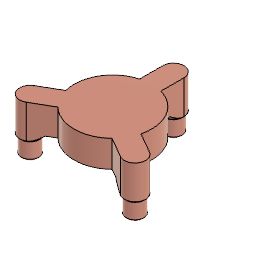
CarrierGenerator (Autodesk Fusion 360 design; units mm, degrees)
Autodesk Fusion 360 part; units mm, degrees
sketch "Sketch5" plane through (0, 0, 0) normal (0, 0, 1) x (1, 0, 0)
  line L0 (0, 0) -> (0, 18) construction
  circle A0 centre (0, 18) radius 2.635
  circle A1 centre (0, 18) radius 3.15
  line L1 (0, 0) -> (2.3742, 0) construction
  circle A2 centre (0, 0) radius 10
  circle A3 centre (0, 0) radius 10.55
  line L2 (0, 18) -> (0, 0) construction
  circle A4 centre (0, 0) radius 11.55
  line L3 (-3.15, 18) -> (-3.15, 11.1122)
  line L4 (3.15, 18) -> (3.15, 11.1122)
  dimension "d167" = 18
  dimension "d168" = 5.27
  dimension "d169" = 6.3
  dimension "d172" = 20
  dimension "d173" = 21.1
  dimension "d177" = 1
  constraint vertical L0
  constraint coincident L0.start L1.start
  constraint coincident L0.end A0.centre
  constraint concentric A0 A1
  constraint perpendicular L0 L1
  constraint concentric A2 A3
  constraint parallel L0 L2
  constraint vertical L3
  constraint coincident A1 L3.start
  constraint coincident A4 L3.end
  constraint tangent A1 L3
  constraint symmetric L0 L3.start L4.start
  constraint symmetric L0 L3.end L4.end
  measures "d167" distance of L0.start L0.end
  measures "d168" diameter of A0
  measures "d169" diameter of A1
  measures "d172" diameter of A2
  measures "d173" diameter of A3
extrude "main body" add sketch "Sketch5" along normal blind 3 contours A4 | A2 | A3
extrude "bearing lip" add sketch "Sketch5" against normal blind 1 contours A3
extrude "wall" add sketch "Sketch5" against normal blind 5 contours A4
fillet "Fillet10" radius 0.5 1 edges at (-9.8361, -3.815, -5)
extrude "planet" add sketch "Sketch5" against normal up to surface (8 mm away) from surface at 3 contours A0 | A1 | A1 A4 L3 L4
extrude "Extrude26" add sketch "Sketch5" against normal blind 2 from surface at -5 contours A0 | A1
extrude "Extrude27" add sketch "Sketch5" against normal blind 5.5 from surface at -7 contours A0
fillet "Fillet8" radius 0.5 1 edges at (-2.4567, 18.9529, -12.5)
chamfer "Chamfer2" distance 0.5 angle 45 1 edges at (-2.4567, 17.0471, -7)
chamfer "Chamfer4" distance 2 angle 45 1 edges at (0, 14.85, -5)
pattern_circular "C-Pattern6" count 3 over 360 about axis through (0, 0, -5) along (0, 0, -1) of "planet", "Extrude26", "Extrude27", "Fillet8", "Chamfer2", "Chamfer4"
sketch "Sketch6" plane through (0, 0, -12.5) normal (0, 0, -1) x (1, 0, 0)
  circle A0 centre (0, -18) radius 2.135
  circle A1 centre (0, -18) radius 1.52
  circle A2 centre (0, 0) radius 18 construction
  dimension "d233" = 3.04
  dimension "d238" = 36
  constraint concentric A0 A1
  constraint coincident A2.centre origin
  measures "d233" diameter of A1
  measures "d238" diameter of A2
extrude "Extrude29" cut sketch "Sketch6" against normal blind 8 contours A1
pattern_circular "C-Pattern7" count 3 over 360 about axis through (0, 0, 3) along (0, 0, 1) of "Extrude29"
equation "gear_ratio = 6"
equation "gear_Ns = 12"
equation "gear_Np = ( gear_ratio - 2 ) * gear_Ns / 2"
equation "planet_carrier_diameter = if(gear_ratio == 6; bearing_4668K225_id; bearing_2349K726_id)"
equation "planet_carrier_width = bearing_4668K225_width"
equation "fit = 0.1 mm"
equation "planets_distance_from_sun = module * ( ( gear_Ns + gear_Np ) / 2 )"
equation "bearing_mount_lip = 1 mm"
equation "thickness = 3 mm"
equation "sun_bearing_od = 21 mm"
equation "sun_bearing_width = 5 mm"
equation "planet_bearing_mount_height = 2 mm"
equation "planet_filet = 0.5 mm"
equation "planet_bearing_clearance = 0.03 mm"
equation "m3 = 3.04 mm"
equation "n_planets = 3" comment "max value is floor(PI/asin(circle_packing))"
equation "d167 = planets_distance_from_sun"
equation "d168 = planet_carrier_diameter - planet_bearing_clearance"
equation "d169 = bearing_mount_lip + planet_carrier_diameter"
equation "d172 = sun_bearing_od - bearing_mount_lip"
equation "d173 = sun_bearing_od + fit"
equation "d197 = thickness"
equation "d203 = -bearing_mount_lip"
equation "d205 = -sun_bearing_width"
equation "d211 = -planet_bearing_mount_height"
equation "d214 = -( planet_carrier_width + planet_filet )"
equation "d220 = planet_filet"
equation "d233 = m3"
equation "d238 = planets_distance_from_sun * 2"
equation "module = 1 mm"
equation "planet_radius = module * ( gear_Np + 2 ) / 2"
equation "circle_packing = planet_radius / planets_distance_from_sun"
equation "bearing_4668K225_id_delta = 0.3 mm"
equation "d260 = n_planets"
equation "m3_length = 10 mm"
equation "d263 = n_planets"
equation "bearing_4668K225_id = 5 mm + bearing_4668K225_id_delta"
equation "bearing_4668K225_width = 5 mm"
equation "bearing_2349K726_id = 12 mm"
